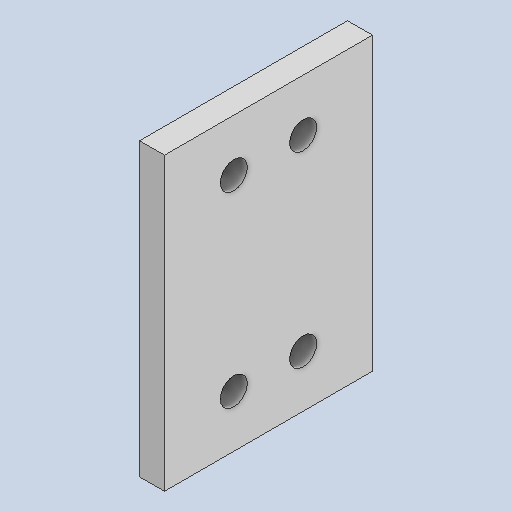
# Autodesk Inventor part: Roter_shaft_support_vertical
Saved by Autodesk Inventor 2026.1 (Build 301233000, 233)
## iProperties
Created: 2025-09-10
Part Number: Roter_shaft_support_vertical
Material: Generic
Document SubType Name: Modeling
Designer: sraav
Density: 1 g/cm^3
Appearance: Default
Author: sraav
Autodesk Inventor part; units mm, degrees
ref_plane "YZ Plane" through (0, 0, 0) normal (1, 0, 0) x (0, 1, 0)
ref_plane "XZ Plane" through (0, 0, 0) normal (0, 1, 0) x (-1, 0, 0)
ref_plane "XY Plane" through (0, 0, 0) normal (0, 0, 1) x (1, 0, 0)
sketch "Sketch1" plane through (0, 0, 0) normal (1, 0, 0) x (0, 1, 0)
  line L0 (0, 0) -> (0, 50)
  line L1 (0, 50) -> (70, 50)
  line L2 (70, 50) -> (70, 0)
  line L3 (70, 0) -> (0, 0)
  circle A0 centre (57.5, 16.6667) radius 3.25
  circle A1 centre (57.5, 33.3333) radius 3.25
  circle A2 centre (12.5, 33.3333) radius 3.25
  circle A3 centre (12.5, 16.6667) radius 3.25
  dimension "d0" = 50
  dimension "d1" = 70
  dimension "d2" = 6.5
  dimension "d3" = 6.5
  dimension "d4" = 6.5
  dimension "d5" = 6.5
  constraints: 8 end point, 4 centre point, 2 perpendicular, 1 horizontal, 1 vertical
  measures "d0" distance of L0.start L0.end
  measures "d1" distance of L0.end L1.end
  measures "d2" diameter of A0
  measures "d3" diameter of A1
  measures "d4" diameter of A2
  measures "d5" diameter of A3
extrude "Extrusion1" add sketch "Sketch1" along normal blind 6
body "Solid1"
